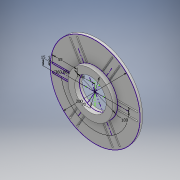
# Autodesk Inventor part: rotor
Saved by Autodesk Inventor 2018 (Build 220112000, 112)
## iProperties
Created: 2024-05-02
Part Number: rotor
Material: Generic
Document SubType Name: Modeling
Designer: neo
Density: 1 g/cm^3
Appearance: Default
Author: neo
Autodesk Inventor part; units mm, degrees
ref_plane "YZ Plane" through (0, 0, 0) normal (1, 0, 0) x (0, 1, 0)
ref_plane "XZ Plane" through (0, 0, 0) normal (0, 1, 0) x (-1, 0, 0)
ref_plane "XY Plane" through (0, 0, 0) normal (0, 0, 1) x (1, 0, 0)
sketch "Sketch1" plane through (0, 0, 0) normal (0, 1, 0) x (-1, 0, 0)
  line L0 (0, 30.3953) -> (0, -28.0277)
  circle A0 centre (0, 0) radius 100
  line L1 (95, 10.5) -> (40, 10.5)
  line L2 (40, 10.5) -> (40, 7.5)
  line L3 (40, 7.5) -> (95, 7.5)
  line L4 (95, 7.5) -> (95, 10.5)
  line L5 (95, -10.5) -> (40, -10.5)
  line L6 (40, -10.5) -> (40, -7.5)
  line L7 (40, -7.5) -> (95, -7.5)
  line L8 (95, -7.5) -> (95, -10.5)
  line L9 (0, 0) -> (75.0694, 0)
  line L10 (0, 0) -> (37.5347, 65.012)
  line L11 (0, 0) -> (-37.5347, 65.012)
  line L12 (0, 0) -> (-75.0694, 0)
  line L13 (0, 0) -> (-37.5347, -65.012)
  line L14 (0, 0) -> (37.5347, -65.012)
  circle A1 centre (0, 0) radius 35
  point P0 (20, 0)
  point P1 (10, 17.3205)
  point P2 (-10, 17.3205)
  point P3 (-20, 0)
  point P4 (-10, -17.3205)
  point P5 (10, -17.3205)
  dimension "d0" = 200
  dimension "t" = 3
  dimension "d2" = 55
  dimension "d3" = 40
  dimension "d4" = 15
  dimension "d21" = 360
  dimension "d27" = 70
  constraints: 30 end point, 6 point on line, 3 parallel, 2 centre point, 2 coincident, 2 collinear, 1 horizontal, 1 perpendicular, 1 vertical, 27 other
  measures "d0" diameter of A0
  measures "t" distance of L3.end L1.start
  measures "d2" distance of L1.start L1.end
  measures "d3" horizontal distance of point (0, 0) L2.end
  measures "d4" distance between parallel lines of L3 L7
  measures "d27" diameter of A1
extrude "Extrusion1" add sketch "Sketch1" along normal blind 6 contours A0 | L4 L3 L2 L1 | L5 L6 L7 L8 | L10 A1 L9 | L11 A1 L10 | L12 A1 L11 | L13 A1 L12 | L14 A1 L13 | L9 A1 L14
extrude "Extrusion3" cut sketch "Sketch1" along normal through all contours L4 L3 L2 L1 | L5 L6 L7 L8
pattern_circular "Circular Pattern1" count 6 over 360 about axis through (0, 0, 0) along (0, 1, 0) of "Extrusion3"
extrude "Extrusion5" cut sketch "Sketch1" along normal through all contours L10 A1 L9 | L11 A1 L10 | L12 A1 L11 | L13 A1 L12 | L14 A1 L13 | L9 A1 L14
sketch "Sketch2" plane through (0, 0, 0) normal (0, -1, 0) x (1, 0, 0)
  circle A0 centre (0, 0) radius 50
  dimension "d30" = 100
  constraints: 1 centre point, 1 coincident
  measures "d30" diameter of A0
extrude "Extrusion6" add sketch "Sketch2" along normal blind 10
extrude "Extrusion7" cut sketch "Sketch1" against normal through all contours L10 A1 L9 | L11 A1 L10 | L12 A1 L11 | L13 A1 L12 | L14 A1 L13 | L9 A1 L14
equation "\"d5\" = 2 * t"
equation "\"d9\" = t"
equation "\"d28\" = t"
body "Solid1"
